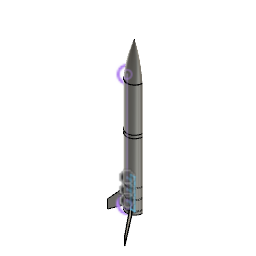
FusionEggRocket (Autodesk Fusion 360 design; units mm, degrees)
Autodesk Fusion 360 part; units mm, degrees
sketch "Sketch4" plane through (0, 0, 0) normal (0, 0, 1) x (1, 0, 0)
  circle A0 centre (0, 0) radius 35
  circle A1 centre (0, 0) radius 34
  dimension "d12" = 70
  dimension "d13" = 68
  constraint coincident A0.centre A1.centre
  constraint concentric A0 A1
  measures "d12" diameter of A0
  measures "d13" diameter of A1
sketch "Sketch5" plane through (0, 0, 0) normal (0, 1, 0) x (1, 0, 0)
  line L0 (-35, 0) -> (35, 0)
  line L1 (35, 0) -> (35, -493)
  line L2 (35, -493) -> (-35, -493)
  line L3 (-35, -493) -> (-35, 0)
  line L4 (0, -493) -> (0, -643)
  spline S0 degree 5 poles (-35, -493) (-34.764, -496.2104) (-34.244, -502.649) (-33.3195, -512.3605) (-31.7933, -525.418) (-29.3702, -541.9005) (-26.4064, -558.4558) (-22.8992, -574.8947) (-18.8987, -590.8567) (-14.5465, -605.7917) (-9.923, -619.5287) (-6.0505, -629.52) (-3.0586, -636.4688) (-1.0259, -640.8627) (0, -643) knots 0 0 0 0 0 0 0.1 0.2 0.3 0.4 0.5 0.6 0.7 0.8 0.9 1 1 1 1 1 1
  line L5 (-25.4293, -564.1284) -> (-17.3308, -597.1289)
  line L6 (0, 0) -> (-33, 0)
  line L7 (-33, 0) -> (-33, -493)
  line L8 (-33, -493) -> (0, -493)
  line L9 (0, -493) -> (0, 0)
  line L10 (-33, -290) -> (35, -290)
  line L11 (-35, 0) -> (35, 0)
  line L12 (-35, -303) -> (35, -303)
  line L13 (-33, -290) -> (-35, -290)
  point P0 (-21.3801, -580.6286)
  dimension "d14" = 70
  dimension "d15" = 493
  dimension "d16" = 150
  dimension "d21" = 290
  dimension "d22" = 303
  dimension "d27" = 33
  constraint horizontal L0
  constraint vertical L1
  constraint horizontal L2
  constraint vertical L3
  constraint midpoint L2 L4.start
  constraint perpendicular L2 L4
  constraint midpoint P0 L5
  constraint horizontal L6
  constraint vertical L7
  constraint horizontal L8
  constraint vertical L9
  constraint coincident L2 L7.end
  constraint coincident L6.start L9.end
  constraint coincident L7 L10.start
  constraint coincident L1 L10.end
  constraint perpendicular L1 L10
  constraint coincident L3 L12.start
  constraint coincident L1 L12.end
  constraint perpendicular L1 L12
  constraint coincident L3 L13.end
  constraint perpendicular L3 L13
  measures "d14" distance of L0.start L0.end
  measures "d15" distance of L0.start L2.end
  measures "d16" distance of L4.start L4.end
  measures "d21" distance of L10 L11
  measures "d22" distance of L11 L12
  measures "d27" distance of L7 L9
revolve "Revolve2" add sketch "Sketch5" angle 360 about axis through (0, 0, 493) along (0, 0, 1) contours L2 L4 S0 L8 makes body 1
shell "Shell1" thickness 2 removed faces 0 bodies 1
revolve "Revolve3" add sketch "Sketch5" angle 360 about axis through (0, 0, 493) along (0, 0, -1) separate body contours L2 L3 L7 L12 makes body 2
revolve "Revolve4" add sketch "Sketch5" angle 360 about axis through (0, 0, 493) along (0, 0, -1) separate body contours L3 L7 L12 L13 makes body 3
revolve "Revolve5" add sketch "Sketch5" angle 360 about axis through (0, 0, 493) along (0, 0, -1) separate body contours L0 L3 L7 L11 L13 makes body 4
sketch "Sketch8" plane through (0, 0, 0) normal (0, 1, 0) x (1, 0, 0)
  line L0 (35, -290) -> (-35, -290)
  line L1 (35, 0) -> (-35, 0)
  line L2 (-35, 0) -> (-118.218, 60.2371)
  line L3 (-118.218, 60.2371) -> (-118.218, 21.0072)
  line L4 (-118.218, 21.0072) -> (-35, -69.8844)
  line L5 (-35, -69.8844) -> (-35, 0)
  point P0 (-35, 0)
  constraint coincident P0 L1.end
  constraint perpendicular L1 L3
extrude "Extrude1" add sketch "Sketch8" along normal mid plane 1.3 separate body makes body 5
pattern_circular "C-Pattern1" count 3 over 360 about axis through (0, 0, 493) along (0, 0, -1) of bodies 5 makes body 6 at (31.9326, 54.0089, 16.2924) makes body 7 at (30.8068, -54.6589, 16.2924)
sketch "Sketch9" plane through (0, 0, 0) normal (0, 1, 0) x (1, 0, 0)
  line L0 (0, 10) -> (-18.5, 10)
  line L1 (-18.5, 10) -> (-18.5, -120)
  line L2 (-18.5, -120) -> (0, -120)
  line L3 (0, -120) -> (0, 10)
  line L4 (0, 10) -> (-15.2, 10)
  line L5 (-15.2, 10) -> (-15.2, -120)
  line L6 (-15.2, -120) -> (0, -120)
  line L7 (0, -120) -> (0, 10)
  line L8 (-33, 0) -> (-33, -493)
  line L9 (-18.5, -99.2638) -> (-33, -99.2638)
  line L10 (-33, -99.2638) -> (-33, -103.2638)
  line L11 (-33, -103.2638) -> (-18.5, -103.2638)
  line L12 (-18.5, -103.2638) -> (-18.5, -99.2638)
  line L13 (-18.5, -59.2638) -> (-33, -59.2638)
  line L14 (-33, -59.2638) -> (-33, -55.2638)
  line L15 (-33, -55.2638) -> (-18.5, -55.2638)
  line L16 (-18.5, -55.2638) -> (-18.5, -59.2638)
  line L17 (-18.5, -11.2638) -> (-33, -11.2638)
  line L18 (-33, -11.2638) -> (-33, -15.2638)
  line L19 (-33, -15.2638) -> (-18.5, -15.2638)
  line L20 (-18.5, -15.2638) -> (-18.5, -11.2638)
  dimension "d32" = 18.5
  dimension "d33" = 130
  dimension "d34" = 15.2
  dimension "d42" = 40
  dimension "d43" = 40
  constraint horizontal L0
  constraint vertical L1
  constraint horizontal L2
  constraint vertical L3
  constraint horizontal L4
  constraint vertical L5
  constraint horizontal L6
  constraint vertical L7
  constraint coincident L2 L5.end
  constraint horizontal L9
  constraint vertical L10
  constraint horizontal L11
  constraint vertical L12
  constraint coincident L8 L10.end
  constraint coincident L1 L9.start
  constraint horizontal L13
  constraint vertical L14
  constraint horizontal L15
  constraint vertical L16
  constraint coincident L8 L14.end
  constraint coincident L1 L13.start
  constraint horizontal L17
  constraint vertical L18
  constraint horizontal L19
  constraint vertical L20
  constraint coincident L8 L18.end
  constraint coincident L1 L17.start
  measures "d32" distance of L0.start L0.end
  measures "d33" distance of L0.start L2.end
  measures "d34" distance of L0.start L4.end
  measures "d42" distance of L15 L19
  measures "d43" distance of L9 L13
revolve "Revolve8" add sketch "Sketch9" angle 360 about axis through (0, 0, 493) along (0, 0, -1) separate body contours L0 L1 L2 L5 L12 L16 L20 makes body 8
revolve "Revolve9" add sketch "Sketch9" angle 360 about axis through (0, 0, 493) along (0, 0, -1) separate body contours L1 L8 L17 L18 L19 L20 | L1 L8 L9 L10 L11 L12 | L1 L8 L13 L14 L15 L16 makes body 9 at (-28.0438, -1.6395, 99.2638) makes body 10 at (-28.0438, -1.6395, 59.2638) makes body 11 at (-28.0438, -1.6395, 11.2638)
sketch "Sketch6" plane through (0, 0, 0) normal (0, 1, 0) x (1, 0, 0)
named bodies: "Cone", "Payload", "Crush", "Body", "Fins", "Fins (1)", "Fins (2)", "MotorTube", "CenteringRing (2)", "CenteringRing", "CenteringRing (1)"
